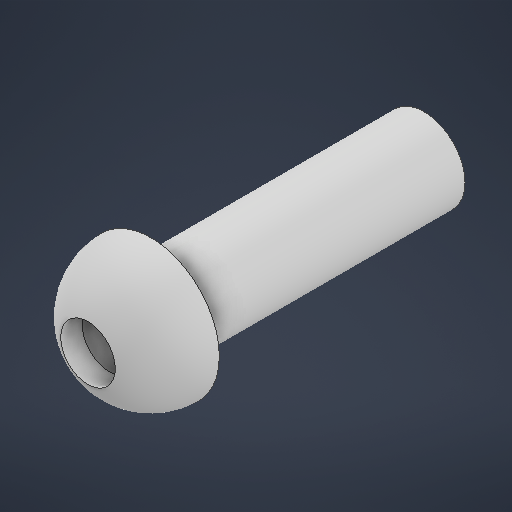
# Autodesk Inventor part: Perno
Saved by Autodesk Inventor 2026.1 (Build 301233020, 233B)
## iProperties
Created: 2025-11-05
Part Number: Perno
Material: Generic
Document SubType Name: Modeling
Designer: Marcelo
Density: 1 g/cm^3
Appearance: Default
Author: Marcelo
Autodesk Inventor part; units mm, degrees
ref_plane "YZ Plane" through (0, 0, 0) normal (1, 0, 0) x (0, 1, 0)
ref_plane "XZ Plane" through (0, 0, 0) normal (0, 1, 0) x (-1, 0, 0)
sketch "Sketch1" plane through (0, 0, 0) normal (0, 0, 1) x (1, 0, 0)
  circle A0 centre (0, 0) radius 1.5
  dimension "d0" = 3
  constraints: 1 centre point, 1 coincident
  measures "d0" diameter of A0
extrude "Extrusion1" add sketch "Sketch1" along normal blind 10
sketch "Sketch2" plane through (0, 0, 0) normal (0, 1, 0) x (-1, 0, 0)
  line L0 (1.5, 10) -> (-1.5, 10) projected
  line L1 (1.5, 0) -> (-1.5, 0) projected
  line L2 (1.5, 10) -> (-1.5, 10) projected
  line L3 (0, 12.0549) -> (0, 7.9451)
  arc A0 (2.5079, 10) -> (-2.5079, 10) centre (0, 10) ccw
  line L4 (-2.5079, 10) -> (2.5079, 10)
  line L5 (0, 10) -> (0, 12.5079)
  point P0 (0, 0)
  constraints: 6 end point, 3 midpoint, 3 point on circle, 1 centre point, 1 coincident, 1 point on line, 1 vertical
revolve "Revolution1" add sketch "Sketch2" angle 360 about axis through (0, 0, 12.0549) along (0, 0, -1) picked at (0.5212, 11.3386) contours L0 L3 L5 A0 L4
ref_plane "Work Plane1" through (0, 0, 12.5079) normal (0, 0, 1) x (1, 0, 0)
sketch "Sketch3" plane through (0, 0, 12.5079) normal (0, 0, 1) x (1, 0, 0)
  circle A0 centre (0, 0) radius 1
  dimension "d4" = 2
  constraints: 1 centre point, 1 coincident
  measures "d4" diameter of A0
extrude "Extrusion2" cut sketch "Sketch3" against normal blind 1
body "Solid1"
